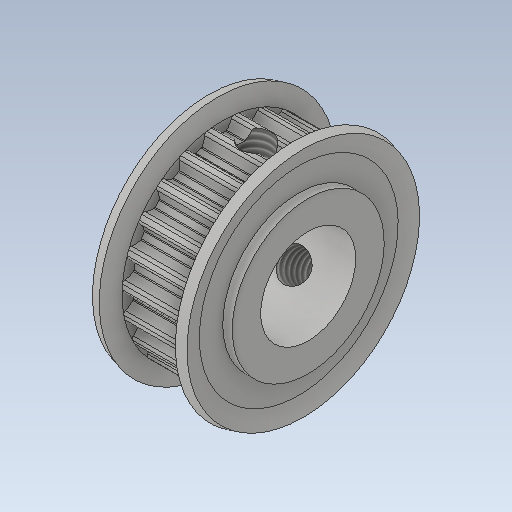
# Autodesk Inventor part: HTPA23S3M060-A-P10_b
Saved by Autodesk Inventor 2020.2 (Build 242310000, 310)
## iProperties
Created: 2022-11-04
Part Number: HTPA23S3M060-A-P10_b
Material: Generic
Catalog Web Link: www.cadenas.de
Description: HTPA__S3M060, HTPA__S3M100, HTPA__S3M150, HTPB__S3M060, HTPB__S3M100, HTPB__S3M150, HTPK__S3M060, HTPK__S3M100, HTPK__S3M150, HTPN__S3M060, HTPN__S3M100, HTPN__S3M150, HTPT__S3M060, HTPT__S3M100, HTPT__S3M150, HTPM__S3M060, HTPM__S3M100, HTPM__S3M150, HTPP__S3M060, HTPP__S3M100, HTPP__S3M150, HTPS__S3M060, HTPS__S3M100, KHTPA__S3M060, KHTPA__S3M100, KHTPA__S3M150, KHTPK__S3M060, KHTPK__S3M100, KHTPK__S3M150_body-High Torque Timing Pulleys S3M Type
Vendor: MISUMI
Document SubType Name: Modeling
Designer: psAdmin
Manufacturer: MISUMI
Mass: 2.63016 g
Surface Area: 24.7129 cm^2
Volume: 2.63016 cm^3
Density: 1 g/cm^3
Appearance: PSOLRGB-175-175-175
Category: PARTsolutions
Company: MISUMI
PSOL_IDENT_0: {$CADENAS_DATA/23d-libs/misumi/metric/51_timing_pulleys/htpk_s3m/htpa_s3m.prj},837 {VTYP=3D},{NB=HTP
PSOL_IDENT_1: A23S3M060-A-P10_b},{LINA=HTPA23S3M060-A-P10},{NN=HTPA__S3M060, HTPA__S3M100, HTPA__S3M150, HTPB__S3M
PSOL_IDENT_2: 060, HTPB__S3M100, HTPB__S3M150, HTPK__S3M060, HTPK__S3M100, HTPK__S3M150, HTPN__S3M060, HTPN__S3M10
PSOL_IDENT_3: 0, HTPN__S3M150, HTPT__S3M060, HTPT__S3M100, HTPT__S3M150, HTPM__S3M060, HTPM__S3M100, HTPM__S3M150,
PSOL_IDENT_4: HTPP__S3M060, HTPP__S3M100, HTPP__S3M150, HTPS__S3M060, HTPS__S3M100, KHTPA__S3M060, KHTPA__S3M100,
PSOL_IDENT_5: KHTPA__S3M150, KHTPK__S3M060, KHTPK__S3M100, KHTPK__S3M150_body},{DATE=28.10.2022 00:10:57},{GEOMDA
PSOL_IDENT_6: TE=11.11.2021 09:52:43},{VERSION=},{LINEID=330},{WBVAR=MATP,ST,TNW,PS,SBS,DD,Z,J,Q,R,S,T,ALT1,ALT2,M
PSOL_IDENT_7: ,QSC,QFC,QTC,ALT3,K,KSC,KFC,KTC,ALT4,ZM,ZSC,ZFC,ZTC,ALT5,ALT6,ALT7,FC,ALT8,SRG,ALT9,BTC,TL,ALT10,TPC
PSOL_IDENT_8: ,ALT11,BC,ALT12,SLH,ALT13,BN},{WBNUMERIC=DD,Z,J,Q,R,S,T,QSC,QFC,QTC,K,KSC,KFC,KTC,ZSC,ZFC,ZTC,FC,SRG
PSOL_IDENT_9: ,BTC,TL,BC,SLH,BN}  {NB=HTPA23S3M060-A-P10_b},{LINA=HTPA23S3M060-A-P10},{KT=DUMMY},{PN=HTPA23S3M060-
PSOL_IDENT_10: A-P10},{TYPE=HTPA},{MATP=A2017},{MATPALG='A2017','Aluminum Alloy 2000 series','S45C','1045 Carbon St
PSOL_IDENT_11: eel Equivalent','SUS304','304 Stainless Steel','A6000','6000 Series Aluminum Alloy'},{ST=CA},{STALG=
PSOL_IDENT_12: 'CA','Clear Anodize','BA','Black Anodize','HAT','Hard Clear Anodize','ENP','Electroless Nickel Plat
PSOL_IDENT_13: ing' },{NT=23},{TNW=S3M060},{TNWALG= 'S3M060','S3M100','S3M150'    },{BW=6},{PS=A},{PSALG='A','B'},{
PSOL_IDENT_14: SBS=P},{SBSALG= 'H','Round Hole','P','Round Hole + Tap','V','Stepped Hole', 'Y','Both Ends Stepped H
PSOL_IDENT_15: ole','WB', 'Double Stepped Hole' },{SHSA= 'H','Round Hole','P','Round Hole + Tap','V','Stepped Hole'
PSOL_IDENT_16: , 'Y','Both Ends Stepped Hole','WB', 'Double Stepped Hole' },{SHSB= 'H','Round Hole','P','Round Hole
PSOL_IDENT_17: + Tap','V','Stepped Hole','F','Stepped Hole (Counterbore holes on the boss side)'},{SHSK='H','Round
PSOL_IDENT_18: Hole','P','Round Hole + Tap'},{SBSPN=-P10},{DD=10.00},{DDALG=[4:4/1],4.5,[5:6/1],6.35,[7:10/1]},{DD
PSOL_IDENT_19: HA=[4:4/1],4.5,[5:6/1],6.35,[7:12/1]},{DDHBK=0},{DDPA=[4:4/1],4.5,[5:6/1],6.35,[7:10/1]},{DDPBK=0},{
PSOL_IDENT_20: DDNA=[8:8/1],[10:11/1]},{DDNBK=0},{DDNK=0},{DDCA=[10:10/1]},{DDCBK=0},{DDVA=[4:4/1],4.5,[5:6/1],6.35
PSOL_IDENT_21: ,[7:10/1]},{DDVF=[4:4/1],4.5,[5:6/1],6.35,[7:8/1]},{DDY=[4:10/1]},{DDWB=[4:8/1]},{Z=0},{ZALG=[0]},{Z
PSOL_IDENT_22: QRMIN=12},{ZAMAX=12},{ZBMAX=10},{DDZ=10},{J=0.0},{JALG=[0]},{JMAX=9},{JMIN=2},{JPN=},{QRMAX=12},{QRM
PSOL_IDENT_23: IN=12},{WBRMAX=-2.00},{WBQMIN=14},{Q=0},{QALG=[0]},{QPN=},{R=0},{RALG=[0]},{S=0.0},{SALG=[0]},{SPN=}
PSOL_IDENT_24: ,{SMAX=5},{T=0.0},{TALG=[0]},{TPN=},{TMAX=8},{A=7},{W=11},{L=0},{PD=21.96},{OD=21.20},{D=0},{DALG=25
PSOL_IDENT_25: },{DE=16},{F=25},{E=16},{BBK=0.000},{TTK=0.0},{TT=1},{ANG=125.217391},{WL=11},{ALT1=},{ALT1ALG= '','
PSOL_IDENT_26: w/o KC90 (Set Screw Angle)','KC90','with KC90 (Set Screw Angle)' },{ALT1PN=},{ALT2=},{ALT2ALG= '','N
PSOL_IDENT_27: ot applicable' },{M=N/A},{MALG= 'N/A' },{MFTALG= 'N/A' },{MSALG= 'N/A' },{M3D=0.000},{KDML=0},{ML=0}
PSOL_IDENT_28: ,{MUL=0},{PITCH=0},{QSC=0.0},{QSCALG=0},{QFC=0.0},{QFCALG=0},{QTC=0.0},{QTCALG=0},{QPCDMIN=0},{QPCDM
PSOL_IDENT_29: INALG=0},{QPCDMAX=12},{ALT2PN=},{ALT3=},{ALT3ALG= '','Not applicable' },{K=0.0},{KALG=0},{KMIN=4},{K
PSOL_IDENT_30: FTMAX=0.0},{KSMAX=0.0},{KSC=0.0},{KSCALG=0},{KFC=0.0},{KFCALG=0},{KTC=0.0},{KTCALG=0},{KPCDMIN=14},{
PSOL_IDENT_31: KPCDMINALG=14},{KPCDMAX=12},{KSCMIN=14.0},{KSCMINALG=14},{ALT3PN=},{ALT4=},{ALT4ALG= '','Not applica
PSOL_IDENT_32: ble' },{ALT4MIN=20.5},{ALT4MAX=5.5},{ZM=N/A},{ZMALG= 'N/A' },{ZMSALG= 'N/A' },{ZMFTALG= 'N/A' },{ZMD
PSOL_IDENT_33: D1=0.0},{ZMDD2=0.0},{ZMHH=0.0},{ZSC=0.0},{ZSCALG=[0]},{ZFC=0.0},{ZFCALG=[0]},{ZTC=0.0},{ZTCALG=[0]},
PSOL_IDENT_34: {ZPCDMIN=0},{ZPCDMINALG=0},{ZPCDMAX=12},{ALT4PN=},{ALT5=},{ALT5ALG= '','Flange Attached','NFC','with
PSOL_IDENT_35: NFC (Flange not Attached)' },{ALT5PN=},{ALT6=},{ALT6ALG= '','w/o Flange Attached on One Side Only','
PSOL_IDENT_36: RFC','with RFC (Flange Attached on The Boss Side Only)','LFC','with LFC (Flange Attached on The Oppo
PSOL_IDENT_37: site Side Only)' },{ALT6PN=},{ALT7=},{ALT7ALG= '','w/o FC (Flange Cut)','FC','with FC (Flange Cut)'
PSOL_IDENT_38: },{FC=0.0},{FCALG=0},{FCMIN=22.5},{FCMAX=23.0},{ALT7PN=},{ALT8=},{ALT8ALG= '','Not applicable' },{AL
PSOL_IDENT_39: T8ALGALG=12},{ALT8DD2=0},{ALT8MM=0},{ALT8NN=0},{QC=0},{KC=0},{ZC=0},{SRG=0.0},{SRGALG=[0]},{SRGMAX1=
PSOL_IDENT_40: 0},{SRGMAX=0},{DD2=0.0},{MM=0.00},{NN=0.00},{ALT8PN=},{ALT9ALG= '','w/o BTC (Taper for Bearing Holde
PSOL_IDENT_41: r)','BTC','with BTC (Taper for Bearing Holder)' },{ALT9=},{BTC9=11},{TL9=1},{BTC=0},{BTCALG=[0]},{TL=
PSOL_IDENT_42: 0.0},{TLALG=0},{TLMIN=1.0},{TLMAX=-11.5},{BTCL=0},{BTCD=0},{BTCDALG=16.000},{ALT9PN=},{WLBCTL=11},{A
PSOL_IDENT_43: LT10=},{ALT10ALG= '','w/o TPC (Tapped Hole Dimension)','TPC','with TPC (Tapped Hole Dimension)' },{T
PSOL_IDENT_44: PC=N/A},{TPCALG= 'N/A' },{TPCM=4},{ALT10PN=},{ALT11=},{ALT11ALG= '','Not applicable' },{BC=0.0},{BCA
PSOL_IDENT_45: LG=0},{BCMIN=7},{BCMAX=-11.5},{BCPLANE=5.5},{M1WBC=5.5},{ALT11PN=},{ALT12=},{ALT12ALG= '','w/o SLH (
PSOL_IDENT_46: Set Screw Length)','SLH','with SLH (Set Screw Length)' },{SLH=0},{SLHALG=[0]},{ALT12PN=},{AC=M4x3},{
PSOL_IDENT_47: M1=4},{M1L=3},{TAP=0.000},{KYY=5},{KTT=5.6},{PLANE=11},{CD=0},{ALT13=},{ALT13ALG= '', 'Not applicabl
PSOL_IDENT_48: e' },{BN=0.0},{BNALG=0},{BNMIN=-10.5},{BNMAX=-1.0},{ALT13PN=}
NB: HTPA23S3M060-A-P10_b
NN: 0
NT: 23
NBSYN: $PN._b
LINA: HTPA23S3M060-A-P10
CATALOG: Misumi
PN: HTPA23S3M060-A-P10
MATP: Aluminum Alloy 2000 series
ST: Clear Anodize
TNW: S3M060
BW: 6
PS: A
SBS: Round Hole + Tap
DD: 10
Z: 0
J: 0
Q: 0
R: 0
S: 0
T: 0
A: 7
W: 11
L: 0
PD: 21.96
OD: 21.2
D: 0
F: 25
E: 16
TT: 1
ALT1: w/o KC90 (Set Screw Angle)
ALT2: Not applicable
M: N/A
QSC: 0
QFC: 0
QTC: 0
ALT3: Not applicable
K: 0
KSC: 0
KFC: 0
KTC: 0
ALT4: Not applicable
ZM: N/A
ZMDD1: 0
ZMDD2: 0
ZMHH: 0
ZSC: 0
ZFC: 0
ZTC: 0
ALT5: Flange Attached
ALT6: w/o Flange Attached on One Side Only
ALT7: w/o FC (Flange Cut)
FC: 0
ALT8: Not applicable
SRG: 0
DD2: 0
MM: 0
ALT9: w/o BTC (Taper for Bearing Holder)
BTC: 0
TL: 0
BTCL: 0
BTCD: 0
ALT10: w/o TPC (Tapped Hole Dimension)
TPC: N/A
ALT11: Not applicable
BC: 0
ALT12: w/o SLH (Set Screw Length)
SLH: 0
AC: M4x3
ALT13: Not applicable
BN: 0
SUPPLIER: MISUMI
ARTICLENO: HTPA23S3M060-A-P10_b
BOMINFO: HTPA23S3M060-A-P10
CREATOR: CADENAS GmbH
Title: HTPA23S3M060-A-P10
Author: Cadenas PARTsolutions
Comments: High Torque Timing Pulleys S3M Type
Autodesk Inventor part; units mm, degrees
sketch "_____1" plane through (0, 0, 0) normal (0, 0, 1) x (1, 0, 0)
  line L0 (11, 0) -> (0, 0)
  line L1 (0, 0) -> (0, 8)
  line L2 (0, 8) -> (1, 8)
  line L3 (1, 8) -> (1, 10.468348)
  line L4 (1, 10.468348) -> (0.524971, 12.241181)
  line L5 (0.524971, 12.241181) -> (1.490897, 12.5)
  line L6 (1.490897, 12.5) -> (2, 10.6)
  line L7 (2, 10.6) -> (9, 10.6)
  line L8 (9, 10.6) -> (9.509103, 12.5)
  line L9 (9.509103, 12.5) -> (10.475029, 12.241181)
  line L10 (10.475029, 12.241181) -> (10, 10.468348)
  line L11 (10, 10.468348) -> (10, 8)
  line L12 (10, 8) -> (11, 8)
  line L13 (11, 8) -> (11, 0)
  line L14 (11, 0) -> (0, 0)
  constraints: 30 end point
revolve "Revolution1" add sketch "_____1" angle 360 about axis through (11, 0, 0) along (1, 0, 0)
sketch "Sketch2" plane through (11, 0, 0) normal (1, 0, 0) x (0, 0, -1)
  point P0 (0, 0)
hole "Hole1" at (11, 0, 0) direction (-1, 0, 0) diameter 10 depth 11
sketch "_____6" plane through (2, 0, 0) normal (1, 0, 0) x (0, 0, -1)
  circle A0 centre (0, 0) radius 15.6
  arc A1 (-10.588933, 0.484249) -> (-10.375701, 0.199463) centre (-10.309225, 0.471458) ccw
  arc A2 (-9.533963, -0.241614) -> (-10.375701, 0.199463) centre (-10.844593, -1.719069) ccw
  arc A3 (-9.483605, -0.34832) -> (-9.533963, -0.241614) centre (-9.633504, -0.353826) ccw
  arc A4 (-9.483605, -0.34832) -> (-9.442704, -0.946275) centre (0, 0) ccw
  arc A5 (-9.478063, -1.058844) -> (-9.442704, -0.946275) centre (-9.591957, -0.961232) ccw
  arc A6 (-10.251901, -1.61043) -> (-9.478063, -1.058844) centre (-10.977666, 0.226385) ccw
  arc A7 (-10.251901, -1.61043) -> (-10.424369, -1.921598) centre (-10.149008, -1.870839) ccw
  arc A8 (-10.424369, -1.921598) -> (-10.326916, -2.390568) centre (0, 0) ccw
  arc A9 (-10.326916, -2.390568) -> (-10.044757, -2.607264) centre (-10.054129, -2.327421) ccw
  arc A10 (-9.115231, -2.804887) -> (-10.044757, -2.607264) centre (-9.978647, -4.581157) ccw
  arc A11 (-9.037952, -2.89405) -> (-9.115231, -2.804887) centre (-9.180807, -2.939793) ccw
  arc A12 (-9.037952, -2.89405) -> (-8.837241, -3.458796) centre (0, 0) ccw
  arc A13 (-8.840918, -3.57673) -> (-8.837241, -3.458796) centre (-8.976924, -3.513466) ccw
  arc A14 (-9.437244, -4.316641) -> (-8.840918, -3.57673) centre (-10.631662, -2.743748) ccw
  arc A15 (-9.437244, -4.316641) -> (-9.519364, -4.662801) centre (-9.267909, -4.539633) ccw
  arc A16 (-9.519364, -4.662801) -> (-9.298998, -5.088088) centre (0, 0) ccw
  arc A17 (-9.298998, -5.088088) -> (-8.968838, -5.220623) centre (-9.053364, -4.953685) ccw
  arc A18 (-8.020464, -5.160134) -> (-8.968838, -5.220623) centre (-8.37263, -7.103482) ccw
  arc A19 (-7.921995, -5.225141) -> (-8.020464, -5.160134) centre (-8.047211, -5.30773) ccw
  arc A20 (-7.921995, -5.225141) -> (-7.57636, -5.714793) centre (0, 0) ccw
  arc A21 (-7.548082, -5.829346) -> (-7.57636, -5.714793) centre (-7.696113, -5.805122) ccw
  arc A22 (-7.92267, -6.702706) -> (-7.548082, -5.829346) centre (-9.497157, -5.510391) ccw
  arc A23 (-7.92267, -6.702706) -> (-7.908351, -7.058185) centre (-7.699451, -6.871743) ccw
  arc A24 (-7.908351, -7.058185) -> (-7.581416, -7.408247) centre (0, 0) ccw
  arc A25 (-7.581416, -7.408247) -> (-7.227742, -7.446791) centre (-7.381152, -7.212558) ccw
  arc A26 (-6.330856, -7.132677) -> (-7.227742, -7.446791) centre (-6.145654, -9.098975) ccw
  arc A27 (-6.2185, -7.168707) -> (-6.330856, -7.132677) centre (-6.31679, -7.282016) ccw
  arc A28 (-6.2185, -7.168707) -> (-5.753576, -7.546951) centre (0, 0) ccw
  arc A29 (-5.69544, -7.649627) -> (-5.753576, -7.546951) centre (-5.844517, -7.666239) ccw
  arc A30 (-5.820507, -8.591662) -> (-5.69544, -7.649627) centre (-7.658291, -7.868353) ccw
  arc A31 (-5.820507, -8.591662) -> (-5.710812, -8.930096) centre (-5.559961, -8.694207) ccw
  arc A32 (-5.710812, -8.930096) -> (-5.301556, -9.178971) centre (0, 0) ccw
  arc A33 (-5.301556, -9.178971) -> (-4.950598, -9.120666) centre (-5.161514, -8.936508) ccw
  arc A34 (-4.171718, -8.576223) -> (-4.950598, -9.120666) centre (-3.462882, -10.419637) ccw
  arc A35 (-4.053807, -8.580603) -> (-4.171718, -8.576223) centre (-4.117882, -8.716229) ccw
  arc A36 (-4.053807, -8.580603) -> (-3.504074, -8.819386) centre (0, 0) ccw
  arc A37 (-3.420393, -8.902569) -> (-3.504074, -8.819386) centre (-3.55946, -8.958786) ccw
  arc A38 (-3.286664, -9.843414) -> (-3.420393, -8.902569) centre (-5.251444, -9.642755) ccw
  arc A39 (-3.286664, -9.843414) -> (-3.089729, -10.139703) centre (-3.008113, -9.871862) ccw
  arc A40 (-3.089729, -10.139703) -> (-2.628503, -10.268932) centre (0, 0) ccw
  arc A41 (-2.628503, -10.268932) -> (-2.30629, -10.118102) centre (-2.559071, -9.997678) ccw
  arc A42 (-1.703182, -9.383709) -> (-2.30629, -10.118102) centre (-0.523285, -10.967524) ccw
  arc A43 (-1.588462, -9.356115) -> (-1.703182, -9.383709) centre (-1.613569, -9.503999) ccw
  arc A44 (-1.588462, -9.356115) -> (-0.994692, -9.437727) centre (0, 0) ccw
  arc A45 (-0.891671, -9.495249) -> (-0.994692, -9.437727) centre (-1.010414, -9.586901) ccw
  arc A46 (-0.509065, -10.365125) -> (-0.891671, -9.495249) centre (-2.455122, -10.701999) ccw
  arc A47 (-0.509065, -10.365125) -> (-0.239494, -10.597294) centre (-0.233168, -10.317366) ccw
  arc A48 (-0.239494, -10.597294) -> (0.239494, -10.597294) centre (0, 0) ccw
  arc A49 (0.239494, -10.597294) -> (0.509065, -10.365125) centre (0.233168, -10.317366) ccw
  arc A50 (0.891671, -9.495249) -> (0.509065, -10.365125) centre (2.455122, -10.701999) ccw
  arc A51 (0.994692, -9.437727) -> (0.891671, -9.495249) centre (1.010414, -9.586901) ccw
  arc A52 (0.994692, -9.437727) -> (1.588462, -9.356115) centre (0, 0) ccw
  arc A53 (1.703182, -9.383709) -> (1.588462, -9.356115) centre (1.613569, -9.503999) ccw
  arc A54 (2.30629, -10.118102) -> (1.703182, -9.383709) centre (0.523285, -10.967524) ccw
  arc A55 (2.30629, -10.118102) -> (2.628503, -10.268932) centre (2.559071, -9.997678) ccw
  arc A56 (2.628503, -10.268932) -> (3.089729, -10.139703) centre (0, 0) ccw
  arc A57 (3.089729, -10.139703) -> (3.286664, -9.843414) centre (3.008113, -9.871862) ccw
  arc A58 (3.420393, -8.902569) -> (3.286664, -9.843414) centre (5.251444, -9.642755) ccw
  arc A59 (3.504074, -8.819386) -> (3.420393, -8.902569) centre (3.55946, -8.958786) ccw
  arc A60 (3.504074, -8.819386) -> (4.053807, -8.580603) centre (0, 0) ccw
  arc A61 (4.171718, -8.576223) -> (4.053807, -8.580603) centre (4.117882, -8.716229) ccw
  arc A62 (4.950598, -9.120666) -> (4.171718, -8.576223) centre (3.462882, -10.419637) ccw
  arc A63 (4.950598, -9.120666) -> (5.301556, -9.178971) centre (5.161514, -8.936508) ccw
  arc A64 (5.301556, -9.178971) -> (5.710812, -8.930096) centre (0, 0) ccw
  arc A65 (5.710812, -8.930096) -> (5.820507, -8.591662) centre (5.559961, -8.694207) ccw
  arc A66 (5.69544, -7.649627) -> (5.820507, -8.591662) centre (7.658291, -7.868353) ccw
  arc A67 (5.753576, -7.546951) -> (5.69544, -7.649627) centre (5.844517, -7.666239) ccw
  arc A68 (5.753576, -7.546951) -> (6.2185, -7.168707) centre (0, 0) ccw
  arc A69 (6.330856, -7.132677) -> (6.2185, -7.168707) centre (6.31679, -7.282016) ccw
  arc A70 (7.227742, -7.446791) -> (6.330856, -7.132677) centre (6.145654, -9.098975) ccw
  arc A71 (7.227742, -7.446791) -> (7.581416, -7.408247) centre (7.381152, -7.212558) ccw
  arc A72 (7.581416, -7.408247) -> (7.908351, -7.058186) centre (0, 0) ccw
  arc A73 (7.908351, -7.058186) -> (7.92267, -6.702706) centre (7.699451, -6.871743) ccw
  arc A74 (7.548082, -5.829346) -> (7.92267, -6.702706) centre (9.497157, -5.510391) ccw
  arc A75 (7.57636, -5.714793) -> (7.548082, -5.829346) centre (7.696113, -5.805122) ccw
  arc A76 (7.57636, -5.714793) -> (7.921995, -5.225141) centre (0, 0) ccw
  arc A77 (8.020464, -5.160134) -> (7.921995, -5.225141) centre (8.047211, -5.30773) ccw
  arc A78 (8.968838, -5.220623) -> (8.020464, -5.160134) centre (8.37263, -7.103482) ccw
  arc A79 (8.968838, -5.220623) -> (9.298998, -5.088088) centre (9.053364, -4.953685) ccw
  arc A80 (9.298998, -5.088088) -> (9.519364, -4.662801) centre (0, 0) ccw
  arc A81 (9.519364, -4.662801) -> (9.437244, -4.316641) centre (9.267909, -4.539633) ccw
  arc A82 (8.840918, -3.57673) -> (9.437244, -4.316641) centre (10.631662, -2.743748) ccw
  arc A83 (8.837241, -3.458796) -> (8.840918, -3.57673) centre (8.976924, -3.513466) ccw
  arc A84 (8.837241, -3.458796) -> (9.037952, -2.89405) centre (0, 0) ccw
  arc A85 (9.115231, -2.804887) -> (9.037952, -2.89405) centre (9.180807, -2.939793) ccw
  arc A86 (10.044757, -2.607264) -> (9.115231, -2.804887) centre (9.978647, -4.581157) ccw
  arc A87 (10.044757, -2.607264) -> (10.326916, -2.390568) centre (10.054129, -2.327421) ccw
  arc A88 (10.326916, -2.390568) -> (10.424369, -1.921598) centre (0, 0) ccw
  arc A89 (10.424369, -1.921598) -> (10.251901, -1.61043) centre (10.149008, -1.870839) ccw
  arc A90 (9.478063, -1.058844) -> (10.251901, -1.61043) centre (10.977666, 0.226385) ccw
  arc A91 (9.442704, -0.946275) -> (9.478063, -1.058844) centre (9.591957, -0.961232) ccw
  arc A92 (9.442704, -0.946275) -> (9.483605, -0.34832) centre (0, 0) ccw
  arc A93 (9.533963, -0.241614) -> (9.483605, -0.34832) centre (9.633504, -0.353826) ccw
  arc A94 (10.375701, 0.199463) -> (9.533963, -0.241614) centre (10.844593, -1.719069) ccw
  arc A95 (10.375701, 0.199463) -> (10.588933, 0.484249) centre (10.309225, 0.471458) ccw
  arc A96 (10.588933, 0.484249) -> (10.556246, 0.962121) centre (0, 0) ccw
  arc A97 (10.556246, 0.962121) -> (10.306222, 1.215219) centre (10.277402, 0.936706) ccw
  arc A98 (9.412263, 1.537571) -> (10.306222, 1.215219) centre (10.509506, 3.179729) ccw
  arc A99 (9.347845, 1.636427) -> (9.412263, 1.537571) centre (9.495598, 1.662292) ccw
  arc A100 (9.347845, 1.636427) -> (9.225903, 2.223243) centre (0, 0) ccw
  arc A101 (9.245604, 2.339578) -> (9.225903, 2.223243) centre (9.371729, 2.258384) ccw
  arc A102 (9.937128, 2.991397) -> (9.245604, 2.339578) centre (10.906246, 1.270515) ccw
  arc A103 (9.937128, 2.991397) -> (10.065618, 3.323152) centre (9.799734, 3.23537) ccw
  arc A104 (10.065618, 3.323152) -> (9.905214, 3.774484) centre (0, 0) ccw
  arc A105 (9.905214, 3.774484) -> (9.596177, 3.950741) centre (9.643567, 3.67478) ccw
  arc A106 (8.648399, 4.019952) -> (9.596177, 3.950741) centre (9.261905, 5.897247) ccw
  arc A107 (8.559699, 4.097762) -> (8.648399, 4.019952) centre (8.694995, 4.162532) ccw
  arc A108 (8.559699, 4.097762) -> (8.283958, 4.629918) centre (0, 0) ccw
  arc A109 (8.271542, 4.747255) -> (8.283958, 4.629918) centre (8.414895, 4.703099) ccw
  arc A110 (8.761563, 5.561473) -> (8.271542, 4.747255) centre (10.159031, 4.165871) ccw
  arc A111 (8.761563, 5.561473) -> (8.795782, 5.915592) centre (8.56344, 5.759331) ccw
  arc A112 (8.795782, 5.915592) -> (8.519559, 6.30691) centre (0, 0) ccw
  arc A113 (8.519559, 6.30691) -> (8.174427, 6.393254) centre (8.294514, 6.140313) ccw
  arc A114 (7.243123, 6.204192) -> (8.174427, 6.393254) centre (7.32739, 8.177393) ccw
  arc A115 (7.136719, 6.255185) -> (7.243123, 6.204192) centre (7.249523, 6.354055) ccw
  arc A116 (7.136719, 6.255185) -> (6.72763, 6.693213) centre (0, 0) ccw
  arc A117 (6.684016, 6.802849) -> (6.72763, 6.693213) centre (6.833967, 6.799007) ccw
  arc A118 (6.936193, 7.71908) -> (6.684016, 6.802849) centre (8.658368, 6.752263) ccw
  arc A119 (6.936193, 7.71908) -> (6.873603, 8.069299) centre (6.692036, 7.856148) ccw
  arc A120 (6.873603, 8.069299) -> (6.502046, 8.371582) centre (0, 0) ccw
  arc A121 (6.502046, 8.371582) -> (6.146418, 8.361609) centre (6.330294, 8.150446) ccw
  arc A122 (5.300658, 7.928295) -> (6.146418, 8.361609) centre (4.849436, 9.851059) ccw
  arc A123 (5.184442, 7.948689) -> (5.300658, 7.928295) centre (5.266388, 8.074327) ccw
  arc A124 (5.184442, 7.948689) -> (4.672344, 8.260103) centre (0, 0) ccw
  arc A125 (4.600768, 8.353907) -> (4.672344, 8.260103) centre (4.746195, 8.390663) ccw
  arc A126 (4.596397, 9.304198) -> (4.600768, 8.353907) centre (6.515554, 8.837871) ccw
  arc A127 (4.596397, 9.304198) -> (4.44164, 9.624543) centre (4.324314, 9.37031) ccw
  arc A128 (4.44164, 9.624543) -> (4.002307, 9.815373) centre (0, 0) ccw
  arc A129 (4.002307, 9.815373) -> (3.662557, 9.709822) centre (3.896586, 9.556099) ccw
  arc A130 (2.965067, 9.064392) -> (3.662557, 9.709822) centre (2.011822, 10.794118) ccw
  arc A131 (2.847658, 9.052676) -> (2.965067, 9.064392) centre (2.892668, 9.195764) ccw
  arc A132 (2.847658, 9.052676) -> (2.270531, 9.214379) centre (0, 0) ccw
  arc A133 (2.176302, 9.285394) -> (2.270531, 9.214379) centre (2.306419, 9.360023) ccw
  arc A134 (1.915707, 10.199266) -> (2.176302, 9.285394) centre (3.889511, 10.268014) ccw
  arc A135 (1.915707, 10.199266) -> (1.680261, 10.465979) centre (1.635877, 10.189519) ccw
  arc A136 (1.680261, 10.465979) -> (1.205735, 10.531201) centre (0, 0) ccw
  arc A137 (1.205735, 10.531201) -> (0.907061, 10.337901) centre (1.173885, 10.253019) ccw
  arc A138 (0.40957, 9.528225) -> (0.907061, 10.337901) centre (-0.975, 10.936625) ccw
  arc A139 (0.299676, 9.485267) -> (0.40957, 9.528225) centre (0.304413, 9.635192) ccw
  arc A140 (0.299676, 9.485267) -> (-0.299676, 9.485267) centre (0, 0) ccw
  arc A141 (-0.40957, 9.528225) -> (-0.299676, 9.485267) centre (-0.304413, 9.635192) ccw
  arc A142 (-0.907061, 10.337901) -> (-0.40957, 9.528225) centre (0.975, 10.936625) ccw
  arc A143 (-0.907061, 10.337901) -> (-1.205735, 10.531201) centre (-1.173885, 10.253019) ccw
  arc A144 (-1.205735, 10.531201) -> (-1.680261, 10.465979) centre (0, 0) ccw
  arc A145 (-1.680261, 10.465979) -> (-1.915707, 10.199266) centre (-1.635877, 10.189519) ccw
  arc A146 (-2.176302, 9.285394) -> (-1.915707, 10.199266) centre (-3.889511, 10.268014) ccw
  arc A147 (-2.270531, 9.214379) -> (-2.176302, 9.285394) centre (-2.306419, 9.360023) ccw
  arc A148 (-2.270531, 9.214379) -> (-2.847658, 9.052676) centre (0, 0) ccw
  arc A149 (-2.965067, 9.064392) -> (-2.847658, 9.052676) centre (-2.892668, 9.195764) ccw
  arc A150 (-3.662557, 9.709822) -> (-2.965067, 9.064392) centre (-2.011822, 10.794118) ccw
  arc A151 (-3.662557, 9.709822) -> (-4.002307, 9.815373) centre (-3.896586, 9.556099) ccw
  arc A152 (-4.002307, 9.815373) -> (-4.44164, 9.624543) centre (0, 0) ccw
  arc A153 (-4.44164, 9.624543) -> (-4.596397, 9.304198) centre (-4.324314, 9.37031) ccw
  arc A154 (-4.600768, 8.353907) -> (-4.596397, 9.304198) centre (-6.515554, 8.837871) ccw
  arc A155 (-4.672344, 8.260103) -> (-4.600768, 8.353907) centre (-4.746195, 8.390663) ccw
  arc A156 (-4.672344, 8.260103) -> (-5.184442, 7.948689) centre (0, 0) ccw
  arc A157 (-5.300658, 7.928295) -> (-5.184442, 7.948689) centre (-5.266388, 8.074327) ccw
  arc A158 (-6.146418, 8.361609) -> (-5.300658, 7.928295) centre (-4.849436, 9.851059) ccw
  arc A159 (-6.146418, 8.361609) -> (-6.502046, 8.371583) centre (-6.330294, 8.150446) ccw
  arc A160 (-6.502046, 8.371583) -> (-6.873603, 8.069299) centre (0, 0) ccw
  arc A161 (-6.873603, 8.069299) -> (-6.936193, 7.71908) centre (-6.692036, 7.856148) ccw
  arc A162 (-6.684016, 6.802849) -> (-6.936193, 7.71908) centre (-8.658368, 6.752263) ccw
  arc A163 (-6.72763, 6.693213) -> (-6.684016, 6.802849) centre (-6.833967, 6.799007) ccw
  arc A164 (-6.72763, 6.693213) -> (-7.136719, 6.255185) centre (0, 0) ccw
  arc A165 (-7.243123, 6.204192) -> (-7.136719, 6.255185) centre (-7.249523, 6.354055) ccw
  arc A166 (-8.174427, 6.393254) -> (-7.243123, 6.204192) centre (-7.32739, 8.177393) ccw
  arc A167 (-8.174427, 6.393254) -> (-8.519559, 6.30691) centre (-8.294514, 6.140313) ccw
  arc A168 (-8.519559, 6.30691) -> (-8.795782, 5.915592) centre (0, 0) ccw
  arc A169 (-8.795782, 5.915592) -> (-8.761563, 5.561473) centre (-8.56344, 5.759331) ccw
  arc A170 (-8.271542, 4.747255) -> (-8.761563, 5.561473) centre (-10.159031, 4.165871) ccw
  arc A171 (-8.283958, 4.629918) -> (-8.271542, 4.747255) centre (-8.414895, 4.703099) ccw
  arc A172 (-8.283958, 4.629918) -> (-8.559699, 4.097762) centre (0, 0) ccw
  arc A173 (-8.648399, 4.019952) -> (-8.559699, 4.097762) centre (-8.694995, 4.162532) ccw
  arc A174 (-9.596177, 3.950741) -> (-8.648399, 4.019952) centre (-9.261905, 5.897247) ccw
  arc A175 (-9.596177, 3.950741) -> (-9.905214, 3.774484) centre (-9.643567, 3.67478) ccw
  arc A176 (-9.905214, 3.774484) -> (-10.065618, 3.323152) centre (0, 0) ccw
  arc A177 (-10.065618, 3.323152) -> (-9.937128, 2.991397) centre (-9.799734, 3.23537) ccw
  arc A178 (-9.245604, 2.339578) -> (-9.937128, 2.991397) centre (-10.906246, 1.270515) ccw
  arc A179 (-9.225903, 2.223243) -> (-9.245604, 2.339578) centre (-9.371729, 2.258384) ccw
  arc A180 (-9.225903, 2.223243) -> (-9.347845, 1.636427) centre (0, 0) ccw
  arc A181 (-9.412263, 1.537571) -> (-9.347845, 1.636427) centre (-9.495598, 1.662292) ccw
  arc A182 (-10.306222, 1.215219) -> (-9.412263, 1.537571) centre (-10.509506, 3.179729) ccw
  arc A183 (-10.306222, 1.215219) -> (-10.556246, 0.962121) centre (-10.277402, 0.936706) ccw
  arc A184 (-10.556246, 0.962121) -> (-10.588933, 0.484249) centre (0, 0) ccw
  constraints: 368 point on circle, 185 centre point
extrude "Extrusion1" cut sketch "_____6" along normal blind 7
sketch "_____18" plane through (5.5, 0, 0) normal (1, 0, 0) x (0, 0, -1)
  line L0 (0, 0) -> (0, 10.6)
  line L1 (0, 10.6) -> (1.621, 10.6)
  line L2 (1.621, 10.6) -> (1.621, 0)
  line L3 (1.621, 0) -> (0, 0)
  line L4 (0, 0) -> (0, 10.6)
  constraints: 10 end point
revolve "Revolution2" cut sketch "_____18" angle 360 about axis through (5.5, 0, 0) along (0, -1, 0)
thread "Thread1" size "M4x0.7" class "6H" standard "ISO Metric profile" length 5.6
sketch "_____19" plane through (5.5, 0, 0) normal (1, 0, 0) x (0, 0, -1)
  line L0 (0, 0) -> (8.659881, -6.112811)
  line L1 (8.659881, -6.112811) -> (7.725082, -7.43712)
  line L2 (7.725082, -7.43712) -> (-0.934799, -1.324308)
  line L3 (-0.934799, -1.324308) -> (0, 0)
  line L4 (0, 0) -> (8.659881, -6.112811)
  constraints: 10 end point
revolve "Revolution3" cut sketch "_____19" angle 360 about axis through (5.5, 0, 0) along (0, 0.5766803, 0.8169699)
thread "Thread2" size "M4x0.7" class "6H" standard "ISO Metric profile" length 5.6 offset 0.1454
ref_plane "to_belt_XY" through (5.5, 0, 0) normal (-1, 0, 0) x (0, 0, -1)
ref_plane "to_belt_YZ" through (5.5, 0, 0) normal (0, 0, -1) x (0, -1, 0)
ref_plane "to_belt_ZX" through (5.5, 0, 0) normal (0, -1, 0) x (-1, 0, 0)
ref_plane "to_screw1_XY" through (5.5, 5, 0) normal (0, 1, 0) x (1, 0, 0)
ref_plane "to_screw1_YZ" through (5.5, 5, 0) normal (1, 0, 0) x (0, 0, -1)
ref_plane "to_screw1_ZX" through (5.5, 5, 0) normal (0, 0, -1) x (0, 1, 0)
ref_plane "to_screw2_XY" through (5.5, -2.883402, -4.084849) normal (0, -0.5766803, -0.8169699) x (1, 0, 0)
ref_plane "to_screw2_YZ" through (5.5, -2.883402, -4.084849) normal (1, 0, 0) x (0, -0.8169699, 0.5766803)
ref_plane "to_screw2_ZX" through (5.5, -2.883402, -4.084849) normal (0, -0.8169699, 0.5766803) x (0, -0.5766803, -0.8169699)
body "Solid1"
